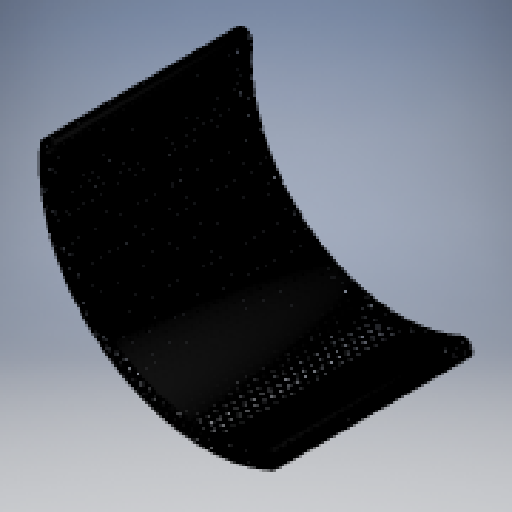
# Autodesk Inventor part: Mesh
Saved by Autodesk Inventor 2026.1 (Build 301233000, 233)
## iProperties
Created: 2025-09-20
Part Number: Mesh
Material: Generic
Document SubType Name: Modeling
Designer: Teddy
Density: 1 g/cm^3
Appearance: Stainless - Satin Coarse Screen
Author: Teddy
Autodesk Inventor part; units mm, degrees
ref_plane "YZ Plane" through (0, 0, 0) normal (1, 0, 0) x (0, 1, 0)
ref_plane "Work Plane1" through (14.1026, -8.3728, 0) normal (0, 0, 1) x (0.9999, -0.0156, 0)
sketch "Sketch1" plane through (14.1026, -8.3728, 0) normal (0, 0, 1) x (0.9999, -0.0156, 0)
  circle A0 centre (-133.5116, -35.2578) radius 2.794 projected
  circle A1 centre (-7.1362, -123.2288) radius 2.286 construction
  circle A2 centre (-67.2141, -131.9038) radius 3.9624 construction
  circle A3 centre (-44.9289, -42.7619) radius 2.286 projected
  arc A4 (-133.5116, -35.2578) -> (-7.1362, -123.2288) centre (-44.9289, -42.7619) ccw construction
  arc A5 (-113.6145, -38.2305) -> (-113.6145, -38.2305) centre (-133.5116, -35.2578) ccw
  arc A6 (-5.1205, -129.2504) -> (-5.1205, -129.2504) centre (-7.1362, -123.2288) ccw
  arc A7 (-133.5116, -35.2578) -> (-7.1362, -123.2288) centre (-44.9289, -42.7619) ccw construction
  arc A8 (-138.5735, -34.829) -> (-4.9766, -127.8269) centre (-44.9289, -42.7619) ccw
  arc A9 (-128.4497, -35.6866) -> (-9.2958, -118.6307) centre (-44.9289, -42.7619) ccw
  arc A10 (-128.4497, -35.6866) -> (-138.5735, -34.829) centre (-133.5116, -35.2578) ccw
  arc A11 (-4.9766, -127.8269) -> (-9.2958, -118.6307) centre (-7.1362, -123.2288) ccw
  point P0 (-14.2313, 8.1521)
  dimension "d0" = 12.7
  dimension "d3" = 10.16
  constraints: 16 point on circle, 8 centre point, 4 tangent, 1 coincident, 1 concentric
  measures "d0" diameter of A6
  measures "d3" diameter of A10
ref_plane "Work Plane2" through (-268.3983, -269.3131, 111.1682) normal (0, 0, -1) x (0, 1, 0)
extrude "Extrusion1" add sketch "Sketch1" along normal up to surface (111.1682 mm away) contours A8 A10 A9 A5 | A5 A9 A6 A8 | A6 A9 A11 A8 picked at (-134.0145, -50.6087) picked at (-9.8396, -124.4417)
body "Solid1"
